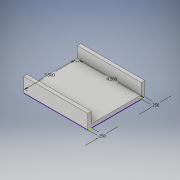
# Autodesk Inventor part: marker relese plate
Saved by Autodesk Inventor 2019 (Build 230136000, 136)
## iProperties
Created: 2018-11-17
Part Number: marker relese plate
Material: Generic
Document SubType Name: Modeling
Designer: User
Density: 1 g/cm^3
Appearance: Default
Author: User
Autodesk Inventor part; units mm, degrees
ref_plane "YZ Plane" through (0, 0, 0) normal (1, 0, 0) x (0, 1, 0)
ref_plane "XZ Plane" through (0, 0, 0) normal (0, 1, 0) x (-1, 0, 0)
ref_plane "XY Plane" through (0, 0, 0) normal (0, 0, 1) x (1, 0, 0)
sketch "Sketch1" plane through (0, 0, 0) normal (0, 1, 0) x (-1, 0, 0)
  line L0 (0, 0) -> (114.3, 0)
  line L1 (114.3, 0) -> (114.3, -88.9)
  line L2 (114.3, -88.9) -> (0, -88.9)
  line L3 (0, -88.9) -> (0, 0)
  line L4 (114.3, 0) -> (0, 0)
  line L5 (0, 0) -> (0, 6.35)
  line L6 (0, 6.35) -> (114.3, 6.35)
  line L7 (114.3, 6.35) -> (114.3, 0)
  line L8 (114.3, -88.9) -> (0, -88.9)
  line L9 (0, -88.9) -> (0, -95.25)
  line L10 (0, -95.25) -> (114.3, -95.25)
  line L11 (114.3, -95.25) -> (114.3, -88.9)
  dimension "d0" = 114.3
  dimension "d1" = 88.9
  dimension "d2" = 6.35
  dimension "d3" = 6.35
  constraints: 24 end point, 6 parallel, 3 horizontal, 3 perpendicular, 1 point on line
  measures "d0" distance of L1.end L2.end
  measures "d1" distance of L0.end L1.end
  measures "d2" distance of L4.end L5.end
  measures "d3" distance of L9.end L8.end
extrude "Extrusion1" add sketch "Sketch1" along normal blind 6.35 contours L0 L1 L2 L3
extrude "Extrusion2" add sketch "Sketch1" along normal blind 25.4 contours L5 L6 L7 L0 | L2 L11 L10 L9
body "Solid1"
